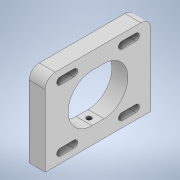
# Autodesk Inventor part: Z_Motorhalter_oben
Saved by Autodesk Inventor 2021.3 (Build 253353000, 353)
## iProperties
Created: 2021-04-21
Part Number: Z_Motorhalter_oben
Material: Generic
Document SubType Name: Modeling
Designer: Fabijan_Sven
Density: 1 g/cm^3
Appearance: Default
Author: Fabijan_Sven
Autodesk Inventor part; units mm, degrees
ref_plane "YZ Plane" through (0, 0, 0) normal (1, 0, 0) x (0, 1, 0)
ref_plane "XZ Plane" through (0, 0, 0) normal (0, 1, 0) x (-1, 0, 0)
ref_plane "XY Plane" through (0, 0, 0) normal (0, 0, 1) x (1, 0, 0)
sketch "Sketch1" plane through (0, 0, 0) normal (0, 1, 0) x (-1, 0, 0)
  line L0 (0, 0) -> (-8, 0)
  line L1 (-8, 0) -> (-8, -27)
  line L2 (-8, -27) -> (0, -27)
  line L3 (0, -27) -> (0, 0)
  line L4 (0, 0) -> (-8, 0)
  line L5 (-8, 0) -> (-8, 26)
  line L6 (-8, 26) -> (0, 26)
  line L7 (0, 26) -> (0, 0)
  dimension "d0" = 8
  dimension "d3" = 27
  dimension "d4" = 26
  constraints: 16 end point, 4 parallel, 2 horizontal, 2 perpendicular, 1 collinear
  measures "d0" distance of L0.start L0.end
  measures "d3" distance between parallel lines of L0 L2
  measures "d4" distance of L6.end L0.start
extrude "Extrusion1" add sketch "Sketch1" along normal blind 41
sketch "Sketch2" plane through (8, 0, 26) normal (1, 0, 0) x (0, 0, -1)
  circle A0 centre (26.5, 20.5) radius 7.5 projected
  circle A1 centre (11, 36) radius 1.5 projected
  circle A2 centre (11, 5) radius 1.5 projected
  circle A3 centre (42, 36) radius 1.5 projected
  circle A4 centre (42, 5) radius 1.5 projected
  arc A5 (14.5, 34.25) -> (14.5, 37.75) centre (14.5, 36) ccw
  arc A6 (7.5, 37.75) -> (7.5, 34.25) centre (7.5, 36) ccw
  line L0 (2.4202, 36) -> (21.3421, 36) construction
  arc A7 (23.5, 32.5) -> (23.5, 8.5) centre (23.5, 20.5) ccw
  arc A8 (29.5, 8.5) -> (29.5, 32.5) centre (29.5, 20.5) ccw
  line L1 (12.5, 20.5) -> (42, 20.5) construction
  line L2 (26.5, 35.5013) -> (26.5, 5.593) construction
  circle A9 centre (42, 36) radius 1.5
  arc A10 (38.5, 37.75) -> (38.5, 34.25) centre (38.5, 36) ccw
  arc A11 (45.5, 34.25) -> (45.5, 37.75) centre (45.5, 36) ccw
  line L3 (45.5, 37.75) -> (38.5, 37.75)
  line L4 (38.5, 34.25) -> (45.5, 34.25)
  circle A12 centre (11, 5) radius 1.5
  circle A13 centre (42, 5) radius 1.5
  arc A14 (14.5, 3.25) -> (14.5, 6.75) centre (14.5, 5) ccw
  arc A15 (7.5, 6.75) -> (7.5, 3.25) centre (7.5, 5) ccw
  line L5 (7.5, 3.25) -> (14.5, 3.25)
  line L6 (14.5, 6.75) -> (7.5, 6.75)
  line L7 (2.4202, 5) -> (21.3421, 5) construction
  circle A16 centre (42, 5) radius 1.5
  arc A17 (38.5, 6.75) -> (38.5, 3.25) centre (38.5, 5) ccw
  line L8 (38.5, 6.75) -> (45.5, 6.75)
  line L9 (45.5, 3.25) -> (38.5, 3.25)
  arc A18 (45.5, 3.25) -> (45.5, 6.75) centre (45.5, 5) ccw
  line L10 (23.5, 32.5) -> (29.5, 32.5)
  line L11 (23.5, 8.5) -> (29.5, 8.5)
  line L12 (7.5, 37.75) -> (14.5, 37.75)
  line L13 (14.5, 34.25) -> (7.5, 34.25)
  point P0 (26, 0)
  point P1 (50.5798, 36)
  point P2 (26.5, 5.4987)
  point P3 (50.5798, 5)
  point P4 (11, 3.5)
  point P5 (11, 6.5)
  point P6 (42, 6.5)
  point P7 (42, 3.5)
  point P8 (42, 37.5)
  point P9 (42, 34.5)
  dimension "d8" = 3.5
  dimension "d9" = 3.5
  dimension "d10" = 3.5
  dimension "d11" = 3.5
  dimension "d14" = 3
  dimension "d15" = 3
  dimension "d16" = 12
  dimension "d17" = 12
  dimension "d33" = 3.5
  constraints: 28 end point, 27 symmetric about line, 20 point on circle, 14 centre point, 9 point on line, 4 horizontal, 2 parallel, 2 tangent, 1 vertical, 10 other
  measures "d8" diameter of A6
  measures "d9" diameter of A5
  measures "d10" distance of A6.centre A1.centre
  measures "d11" distance of A1.centre A5.centre
  measures "d14" distance of A8.centre A0.centre
  measures "d15" distance of A0.centre A7.centre
  measures "d16" radius of A7
  measures "d17" radius of A8
  measures "d33" distance between parallel lines of L13 L12
extrude "Extrusion2" cut sketch "Sketch2" against normal blind 10 contours A0 | A1 | A2 | A3 | A4 | L13 A6 L12 A5 | L10 A8 L11 A7 | L3 A11 L4 A10 | L5 A15 L6 A14 | L8 A18 L9 A17
fillet "Fillet1" radius 5 2 edges at (4, 41, 26) (4, 41, -27)
sketch "Sketch3" plane through (0, 0, 0) normal (0, -1, 0) x (1, 0, 0)
  line L0 (4, 28.9228) -> (4, -37.7056) construction
  circle A0 centre (4, 22) radius 1.5
  circle A1 centre (4, -23) radius 1.5
  circle A2 centre (4, 0) radius 1.5
  line L1 (8, 26) -> (8, -27) projected
  line L2 (0, 26) -> (8, 26) projected
  line L3 (8, -27) -> (0, -27) projected
  point P0 (0, 0)
  dimension "d20" = 3
  dimension "d21" = 3
  dimension "d22" = 3
  dimension "d23" = 4
  dimension "d24" = 4
  dimension "d25" = 4
  constraints: 3 centre point, 3 point on line, 2 end point, 1 vertical
  measures "d20" diameter of A0
  measures "d21" diameter of A2
  measures "d22" diameter of A1
  measures "d23" distance between parallel lines of L1 L0
  measures "d24" distance from line of L2 A0.centre
  measures "d25" distance from line of L3 A1.centre
hole "Hole2" at (4, 0, 22) at (4, 0, 0) at (4, 0, -23) direction (0, 1, 0) diameter 2.459 depth 20 tip angle 118 thread size "M3x0.5" class "6H" standard "ISO Metric profile"
body "Solid1"
